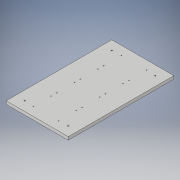
# Autodesk Inventor part: Assembly Plate
Saved by Autodesk Inventor 2019.4 (Build 234330000, 330)
## iProperties
Created: 2021-01-11
Part Number: Assembly Plate
Material: Generic
Document SubType Name: Modeling
Designer: caleb
Density: 1 g/cm^3
Appearance: Default
Author: caleb
Autodesk Inventor part; units mm, degrees
ref_plane "YZ Plane" through (0, 0, 0) normal (1, 0, 0) x (0, 1, 0)
ref_plane "XZ Plane" through (0, 0, 0) normal (0, 1, 0) x (-1, 0, 0)
ref_plane "XY Plane" through (0, 0, 0) normal (0, 0, 1) x (1, 0, 0)
sketch "Sketch1" plane through (0, 0, 0) normal (0, 1, 0) x (-1, 0, 0)
  line L0 (-63.5, 107.95) -> (63.5, 107.95)
  line L1 (63.5, 107.95) -> (63.5, -107.95)
  line L2 (63.5, -107.95) -> (-63.5, -107.95)
  line L3 (-63.5, -107.95) -> (-63.5, 107.95)
  line L4 (-63.5, 107.95) -> (63.5, -107.95) construction
  line L5 (63.5, 107.95) -> (-63.5, -107.95) construction
  point P0 (0, 0)
  dimension "d0" = 127
  dimension "d1" = 215.9
  constraints: 12 end point, 2 midpoint, 2 parallel, 1 horizontal, 1 perpendicular
  measures "d0" distance of L1.end L2.end
  measures "d1" distance of L0.end L1.end
extrude "Extrusion1" add sketch "Sketch1" along normal blind 6.35
sketch "Sketch2" plane through (0, 6.35, 0) normal (0, 1, 0) x (1, 0, 0)
  line L0 (-63.5, -107.95) -> (63.5, -107.95) projected
  line L1 (-63.5, 107.95) -> (-63.5, -107.95) projected
  circle A0 centre (-25.7556, -89.8347) radius 1.25
  circle A1 centre (-25.7556, -53.7347) radius 1.25
  circle A2 centre (25.7444, -89.8347) radius 1.25
  circle A3 centre (25.7444, -53.7347) radius 1.25
  circle A4 centre (-25.7556, -41.976) radius 1.25
  circle A5 centre (-25.7556, -5.876) radius 1.25
  circle A6 centre (25.7444, -41.976) radius 1.25
  circle A7 centre (25.7444, -5.876) radius 1.25
  circle A8 centre (-25.7556, 5.8826) radius 1.25
  circle A9 centre (-25.7556, 41.9826) radius 1.25
  circle A10 centre (25.7444, 5.8826) radius 1.25
  circle A11 centre (25.7444, 41.9826) radius 1.25
  circle A12 centre (-25.7556, 53.7413) radius 1.25
  circle A13 centre (-25.7556, 89.8413) radius 1.25
  circle A14 centre (25.7444, 53.7413) radius 1.25
  circle A15 centre (25.7444, 89.8413) radius 1.25
  point P0 (0, 0)
  dimension "d5" = 18.1153
  dimension "d6" = 37.7444
  dimension "d7" = 2.5
  dimension "d8" = 2.5
  dimension "d9" = 36.1
  dimension "d10" = 2.5
  dimension "d11" = 51.5
  dimension "d12" = 2.5
  dimension "d15" = 47.8587
  constraints: 16 centre point, 2 horizontal alignment, 2 vertical alignment, 1 vertical, 24 other
  measures "d5" distance from line of L0 A0.centre
  measures "d6" distance from line of L1 A0.centre
  measures "d7" diameter of A0
  measures "d8" diameter of A1
  measures "d9" distance of A1.centre A0.centre
  measures "d10" diameter of A2
  measures "d11" distance of A2.centre A0.centre
  measures "d12" diameter of A3
  measures "d15" distance of A0.centre A4.centre
hole "Hole1" at (-25.7556, 6.35, 89.8347) at (25.7444, 6.35, 89.8347) at (25.7444, 6.35, 53.7347) at (-25.7556, 6.35, 53.7347) at (-25.7556, 6.35, 41.976) at (25.7444, 6.35, 41.976) at (25.7444, 6.35, 5.876) at (-25.7556, 6.35, 5.876) at (-25.7556, 6.35, -5.8826) at (25.7444, 6.35, -5.8826) at (25.7444, 6.35, -41.9826) at (-25.7556, 6.35, -41.9826) at (-25.7556, 6.35, -53.7413) at (25.7444, 6.35, -53.7413) at (25.7444, 6.35, -89.8413) at (-25.7556, 6.35, -89.8413) direction (0, -1, 0) diameter 1.5748 end through all
sketch "Sketch5" plane through (0, 6.35, 0) normal (0, 1, 0) x (1, 0, 0)
  line L0 (-63.5, 107.95) -> (-63.5, -107.95) projected
  line L1 (-63.5, -107.95) -> (63.5, -107.95) projected
  point P0 (0, 0)
  point P1 (-44.45, -88.9)
  point P2 (-44.45, 88.9)
  point P3 (44.45, -88.9)
  point P4 (44.45, 88.9)
  dimension "d36" = 19.05
  dimension "d37" = 19.05
  dimension "d40" = 177.8
  dimension "d43" = 88.9
  constraints: 1 horizontal, 1 vertical, 3 other
  measures "d36" distance from line of L0 point (-44.45, -88.9)
  measures "d37" distance from line of L1 point (-44.45, -88.9)
  measures "d40" distance of point (-44.45, -88.9) point (-44.45, 88.9)
  measures "d43" distance of point (-44.45, -88.9) point (44.45, -88.9)
hole "Hole2" at (-44.45, 6.35, 88.9) at (-44.45, 6.35, -88.9) at (44.45, 6.35, 88.9) at (44.45, 6.35, -88.9) direction (0, -1, 0) diameter 2.4638 end through all
body "Solid1"
